Autodesk Inventor part; units mm, degrees
(part 2 of 2)
  line L683 (13.8193, -16.6595) -> (13.4103, -17.1969)
  line L684 (13.4103, -17.1969) -> (13.0544, -17.8466)
  line L685 (13.0544, -17.8466) -> (12.7817, -18.5147)
  line L686 (12.7817, -18.5147) -> (12.6178, -19.1068)
  line L687 (12.6178, -19.1068) -> (12.5603, -19.6314)
  line L688 (12.5603, -19.6314) -> (12.6069, -20.0971)
  line L689 (12.6069, -20.0971) -> (12.7553, -20.5124)
  line L690 (12.7553, -20.5124) -> (13.0032, -20.8859)
  line L691 (13.0032, -20.8859) -> (13.3484, -21.2261)
  line L692 (13.3484, -21.2261) -> (13.7885, -21.5415)
  line L693 (13.7885, -21.5415) -> (16.5319, -23.0238)
  line L694 (16.5319, -23.0238) -> (20.3466, -25.1761)
  line L695 (20.3466, -25.1761) -> (20.6486, -25.4525)
  line L696 (20.6486, -25.4525) -> (20.8116, -25.7931)
  line L697 (20.8116, -25.7931) -> (20.8459, -26.1675)
  line L698 (20.8459, -26.1675) -> (20.7618, -26.5456)
  line L699 (20.7618, -26.5456) -> (20.5697, -26.8968)
  line L700 (20.5697, -26.8968) -> (20.2799, -27.1909)
  line L701 (20.2799, -27.1909) -> (19.9026, -27.3974)
  line L702 (19.9026, -27.3974) -> (19.4483, -27.4862)
  line L703 (19.4483, -27.4862) -> (17.3984, -27.5067)
  line L704 (17.3984, -27.5067) -> (16.3264, -27.4862)
  line L705 (16.3264, -27.4862) -> (16.0758, -27.4173)
  line L706 (16.0758, -27.4173) -> (15.8933, -27.2387)
  line L707 (15.8933, -27.2387) -> (15.8038, -26.9924)
  line L708 (15.8038, -26.9924) -> (15.8323, -26.7206)
  line L709 (15.8323, -26.7206) -> (15.8735, -26.4369)
  line L710 (15.8735, -26.4369) -> (15.7983, -26.1616)
  line L711 (15.7983, -26.1616) -> (15.592, -25.9517)
  line L712 (15.592, -25.9517) -> (15.2394, -25.864)
  line L713 (15.2394, -25.864) -> (11.0542, -25.864)
  line L714 (11.0542, -25.864) -> (10.6479, -25.9075)
  line L715 (10.6479, -25.9075) -> (10.3167, -26.0305)
  line L716 (10.3167, -26.0305) -> (10.0596, -26.2215)
  line L717 (10.0596, -26.2215) -> (9.8757, -26.4694)
  line L718 (9.8757, -26.4694) -> (9.764, -26.7626)
  line L719 (9.764, -26.7626) -> (9.7235, -27.0899)
  line L720 (9.7235, -27.0899) -> (9.7533, -27.4399)
  line L721 (9.7533, -27.4399) -> (9.8525, -27.8013)
  line L722 (9.8525, -27.8013) -> (10.0202, -28.1626)
  line L723 (10.0202, -28.1626) -> (10.2553, -28.5126)
  line L724 (10.2553, -28.5126) -> (10.5569, -28.8399)
  line L725 (10.5569, -28.8399) -> (10.9242, -29.1332)
  line L726 (10.9242, -29.1332) -> (11.356, -29.381)
  line L727 (11.356, -29.381) -> (11.8516, -29.5721)
  line L728 (11.8516, -29.5721) -> (12.4099, -29.6951)
  line L729 (12.4099, -29.6951) -> (13.03, -29.7386)
  line L730 (13.03, -29.7386) -> (21.965, -29.7386)
  line L731 (21.965, -29.7386) -> (22.6253, -29.702)
  line L732 (22.6253, -29.702) -> (23.2336, -29.5897)
  line L733 (23.2336, -29.5897) -> (23.7942, -29.3979)
  line L734 (23.7942, -29.3979) -> (24.3112, -29.1228)
  line L735 (24.3112, -29.1228) -> (24.7889, -28.7605)
  line L736 (24.7889, -28.7605) -> (25.2316, -28.3073)
  line L737 (25.2316, -28.3073) -> (25.6435, -27.7593)
  line L738 (25.6435, -27.7593) -> (26.0289, -27.1127)
  line L739 (26.0289, -27.1127) -> (26.4193, -26.2607)
  line L740 (26.4193, -26.2607) -> (26.6201, -25.5322)
  line L741 (26.6201, -25.5322) -> (26.6506, -24.9094)
  line L742 (26.6506, -24.9094) -> (26.5304, -24.3745)
  line L743 (26.5304, -24.3745) -> (26.2786, -23.9096)
  line L744 (26.2786, -23.9096) -> (25.9146, -23.4968)
  line L745 (25.9146, -23.4968) -> (25.4579, -23.1183)
  line L746 (25.4579, -23.1183) -> (24.9277, -22.7562)
  line L747 (35.8308, -12.5417) -> (35.6711, -12.3549)
  line L748 (35.6711, -12.3549) -> (35.4659, -12.2167)
  line L749 (35.4659, -12.2167) -> (34.9498, -12.1015)
  line L750 (34.9498, -12.1015) -> (12.9562, -12.1015)
  line L751 (12.9562, -12.1015) -> (12.48, -12.1781)
  line L752 (12.48, -12.1781) -> (12.03, -12.39)
  line L753 (12.03, -12.39) -> (11.6489, -12.7098)
  line L754 (11.6489, -12.7098) -> (11.3795, -13.1102)
  line L755 (11.3795, -13.1102) -> (2.0043, -33.4309)
  line L756 (2.0043, -33.4309) -> (1.8927, -33.9479)
  line L757 (1.8927, -33.9479) -> (1.9323, -34.1923)
  line L758 (1.9323, -34.1923) -> (2.0351, -34.4159)
  line L759 (2.0351, -34.4159) -> (2.1948, -34.6028)
  line L760 (2.1948, -34.6028) -> (2.4002, -34.7412)
  line L761 (2.4002, -34.7412) -> (2.9168, -34.8567)
  line L762 (2.9168, -34.8567) -> (24.9341, -34.8567)
  line L763 (24.9341, -34.8567) -> (25.4106, -34.7799)
  line L764 (25.4106, -34.7799) -> (25.8605, -34.5676)
  line L765 (25.8605, -34.5676) -> (26.2412, -34.2474)
  line L766 (26.2412, -34.2474) -> (26.5102, -33.8467)
  line L767 (26.5102, -33.8467) -> (28.1619, -30.2583)
  line L768 (28.1619, -30.2583) -> (27.8028, -29.9601)
  line L769 (27.8028, -29.9601) -> (27.5106, -29.5935)
  line L770 (27.5106, -29.5935) -> (27.4336, -29.462)
  line L771 (27.4336, -29.462) -> (26.3715, -31.7689)
  line L772 (26.3715, -31.7689) -> (3.8665, -31.7689)
  line L773 (3.8665, -31.7689) -> (12.2831, -13.5267)
  line L774 (12.2831, -13.5267) -> (12.2831, -13.526)
  line L775 (12.2831, -13.526) -> (12.482, -13.0955)
  line L776 (12.482, -13.0955) -> (34.9498, -13.0955)
  line L777 (34.9498, -13.0955) -> (34.9639, -13.0968)
  line L778 (34.9639, -13.0968) -> (34.9594, -13.1109)
  line L779 (34.9594, -13.1109) -> (32.7699, -17.8684)
  line L780 (32.7699, -17.8684) -> (33.3832, -17.6303)
  line L781 (33.3832, -17.6303) -> (34.036, -17.4956)
  line L782 (34.036, -17.4956) -> (35.8629, -13.5267)
  line L783 (35.8629, -13.5267) -> (35.9739, -13.0094)
  line L784 (35.9739, -13.0094) -> (35.934, -12.765)
  line L785 (35.934, -12.765) -> (35.8308, -12.5417)
  point P0 (100, -50)
  point P1 (43.169, -21.3602)
  point P2 (43.426, -20.7976)
  point P3 (38.2792, -20.4356)
  point P4 (38.4651, -20.5971)
  point P5 (44.1555, -29.7302)
  constraints: 1572 end point, 1 point on line
sketch "Sketch17" plane through (-58, 50, -100) normal (-1, 0, 0) x (0, 0, 1)
  arc A0 (155.5169, -13.1936) -> (147.9671, -13.2014) centre (177.9783, -25519.1247) ccw
  arc A1 (164.0422, -13.1874) -> (155.5169, -13.1936) centre (180.5222, -28431.0385) ccw
  arc A2 (172.4068, -13.1839) -> (164.0422, -13.1874) centre (179.3768, -26483.535) ccw
  line L0 (172.4068, -13.1839) -> (192.49, -13.1786)
  line L1 (192.49, -13.1786) -> (192.4714, -13.7779)
  arc A3 (192.4714, -13.7779) -> (192.463, -14.0923) centre (229.4243, -14.9268) ccw
  arc A4 (192.463, -14.0923) -> (192.4526, -14.5768) centre (388.1411, -18.5105) ccw
  arc A5 (192.4526, -14.5768) -> (192.4423, -15.1225) centre (411.7864, -18.9861) ccw
  arc A6 (192.4423, -15.1225) -> (192.4336, -15.6562) centre (393.0535, -18.6562) ccw
  arc A7 (192.4247, -16.1476) -> (192.4336, -15.6562) centre (117.8838, -14.5414) ccw
  arc A8 (192.4135, -16.5636) -> (192.4247, -16.1476) centre (153.9256, -15.3181) ccw
  arc A9 (192.4012, -16.933) -> (192.4135, -16.5636) centre (-72.1561, -8.0018) ccw
  arc A10 (192.3918, -16.9493) -> (192.4012, -16.933) centre (192.3813, -16.9323) ccw
  arc A11 (192.3716, -16.9551) -> (192.3918, -16.9493) centre (192.3711, -16.9157) ccw
  arc A12 (191.4025, -16.9687) -> (192.3716, -16.9551) centre (85.6627, 7554.4624) ccw
  arc A13 (190.3279, -16.9824) -> (191.4025, -16.9687) centre (185.5858, 399.5447) ccw
  arc A14 (189.0559, -16.9958) -> (190.3279, -16.9824) centre (181.0678, 796.3096) ccw
  line L2 (189.0559, -16.9958) -> (185.7427, -17.0284)
  line L3 (185.7427, -17.0284) -> (184.3599, -17.8038)
  arc A15 (183.8287, -18.1011) -> (184.3599, -17.8038) centre (-6.9765, 323.4154) ccw
  arc A16 (183.3793, -18.3514) -> (183.8287, -18.1011) centre (86.1277, 156.7717) ccw
  arc A17 (182.9739, -18.5765) -> (183.3793, -18.3514) centre (-1472.0251, 2962.5768) ccw
  arc A18 (182.9636, -18.5792) -> (182.9739, -18.5765) centre (182.9636, -18.558) ccw
  arc A19 (182.9533, -18.5766) -> (182.9636, -18.5792) centre (182.9636, -18.5575) ccw
  arc A20 (182.535, -18.3501) -> (182.9533, -18.5766) centre (1951.8004, 3249.2088) ccw
  arc A21 (182.0715, -18.0984) -> (182.535, -18.3501) centre (284.7979, 170.5134) ccw
  arc A22 (181.5235, -17.7994) -> (182.0715, -18.0984) centre (382.7242, 350.3106) ccw
  line L4 (181.5235, -17.7994) -> (180.0969, -17.0197)
  line L5 (180.0969, -17.0197) -> (160.1888, -17.0208)
  arc A23 (160.1888, -17.0208) -> (144.3749, -17.0268) centre (161.6341, -24881.6326) ccw
  arc A24 (144.3749, -17.0268) -> (136.8231, -17.0497) centre (145.4933, -1626.5302) ccw
  arc A25 (136.8231, -17.0497) -> (132.0963, -17.0846) centre (143.2266, -1205.9023) ccw
  arc A26 (132.0963, -17.0846) -> (131.0777, -17.1776) centre (132.155, -23.3486) ccw
  arc A27 (131.0777, -17.1776) -> (130.7549, -17.273) centre (131.3311, -18.6291) ccw
  arc A28 (130.7549, -17.273) -> (130.46, -17.4396) centre (131.3448, -18.6615) ccw
  arc A29 (130.46, -17.4396) -> (130.2164, -17.663) centre (131.3024, -18.6028) ccw
  arc A30 (130.2164, -17.663) -> (130.0444, -17.9258) centre (131.1049, -18.4319) ccw
  arc A31 (130.0444, -17.9258) -> (129.9153, -18.3085) centre (131.5687, -18.6533) ccw
  arc A32 (129.9153, -18.3085) -> (129.8325, -18.8421) centre (135.0438, -19.3779) ccw
  arc A33 (129.8325, -18.8421) -> (129.791, -19.5222) centre (137.9858, -19.6803) ccw
  arc A34 (129.791, -19.5222) -> (129.7932, -20.3697) centre (149.1997, -19.8967) ccw
  arc A35 (129.7932, -20.3697) -> (129.8114, -20.9203) centre (161.1402, -19.6056) ccw
  arc A36 (129.8114, -20.9203) -> (129.8371, -21.2992) centre (137.1928, -20.6105) ccw
  arc A37 (129.8371, -21.2992) -> (129.8752, -21.5913) centre (133.8851, -20.9202) ccw
  arc A38 (129.8752, -21.5913) -> (129.932, -21.8528) centre (132.6128, -21.1331) ccw
  arc A39 (129.932, -21.8528) -> (130.0762, -22.1968) centre (131.2735, -21.4927) ccw
  arc A40 (130.0762, -22.1968) -> (130.3004, -22.4677) centre (131.0286, -21.6367) ccw
  arc A41 (130.3004, -22.4677) -> (130.6022, -22.658) centre (131.0525, -21.6094) ccw
  arc A42 (130.6022, -22.658) -> (130.9734, -22.7654) centre (131.2185, -21.223) ccw
  arc A43 (130.9734, -22.7654) -> (131.5045, -22.8166) centre (131.6549, -18.476) ccw
  arc A44 (131.5045, -22.8166) -> (132.8291, -22.855) centre (135.5677, 94.4652) ccw
  arc A45 (132.8291, -22.855) -> (134.8809, -22.8934) centre (138.0008, 198.702) ccw
  arc A46 (134.8809, -22.8934) -> (138.4757, -22.9405) centre (161.0223, 1833.8913) ccw
  arc A47 (141.0206, -22.9772) -> (138.4757, -22.9405) centre (131.717, -579.5957) ccw
  arc A48 (142.6378, -23.0177) -> (141.0206, -22.9772) centre (139.3924, -120.3907) ccw
  arc A49 (143.7571, -23.0692) -> (142.6378, -23.0177) centre (141.1689, -67.087) ccw
  arc A50 (144.5556, -23.1431) -> (143.7571, -23.0692) centre (143.0556, -34.9983) ccw
  arc A51 (145.317, -23.2838) -> (144.5556, -23.1431) centre (143.701, -29.8979) ccw
  arc A52 (146.093, -23.5149) -> (145.317, -23.2838) centre (143.3852, -31.1905) ccw
  arc A53 (146.8189, -23.8134) -> (146.093, -23.5149) centre (143.5298, -30.7805) ccw
  arc A54 (147.4285, -24.1566) -> (146.8189, -23.8134) centre (144.7359, -28.2256) ccw
  arc A55 (147.7255, -24.3826) -> (147.4285, -24.1566) centre (145.8661, -26.5177) ccw
  arc A56 (148.0655, -24.7) -> (147.7255, -24.3826) centre (143.2906, -29.4751) ccw
  arc A57 (148.383, -25.0401) -> (148.0655, -24.7) centre (143.2904, -29.4753) ccw
  arc A58 (148.609, -25.3371) -> (148.383, -25.0401) centre (146.2466, -26.9007) ccw
  arc A59 (148.9308, -25.9) -> (148.609, -25.3371) centre (144.4706, -28.0761) ccw
  arc A60 (149.1657, -26.484) -> (148.9308, -25.9) centre (144.9676, -27.8336) ccw
  arc A61 (149.3254, -27.126) -> (149.1657, -26.484) centre (144.4771, -27.9913) ccw
  arc A62 (149.4214, -27.8641) -> (149.3254, -27.126) centre (141.5782, -28.5088) ccw
  arc A63 (149.4533, -28.4552) -> (149.4214, -27.8641) centre (138.9674, -28.7233) ccw
  arc A64 (149.4702, -29.3971) -> (149.4533, -28.4552) centre (87.0184, -30.052) ccw
  arc A65 (149.4733, -30.3333) -> (149.4702, -29.3971) centre (84.3091, -30.0805) ccw
  arc A66 (149.4529, -30.8676) -> (149.4733, -30.3333) centre (141.6731, -30.3031) ccw
  arc A67 (149.3251, -31.9543) -> (149.4529, -30.8676) centre (137.2306, -29.9807) ccw
  arc A68 (149.1085, -32.8875) -> (149.3251, -31.9543) centre (142.1906, -30.7901) ccw
  arc A69 (148.8006, -33.6818) -> (149.1085, -32.8875) centre (143.7022, -31.2484) ccw
  arc A70 (148.3967, -34.35) -> (148.8006, -33.6818) centre (145.2104, -31.9682) ccw
  arc A71 (147.9836, -34.8205) -> (148.3967, -34.35) centre (145.2057, -31.9647) ccw
  arc A72 (147.4851, -35.2416) -> (147.9836, -34.8205) centre (144.7342, -31.48) ccw
  arc A73 (146.9055, -35.6091) -> (147.4851, -35.2416) centre (144.4327, -31.0677) ccw
  arc A74 (146.2491, -35.9202) -> (146.9055, -35.6091) centre (143.8047, -29.9143) ccw
  arc A75 (145.5174, -36.1782) -> (146.2491, -35.9202) centre (143.1741, -28.3651) ccw
  arc A76 (144.8818, -36.3144) -> (145.5174, -36.1782) centre (144.3529, -32.2955) ccw
  arc A77 (144.0427, -36.3836) -> (144.8818, -36.3144) centre (143.7489, -27.7054) ccw
  arc A78 (142.4034, -36.4263) -> (144.0427, -36.3836) centre (140.5007, 68.2463) ccw
  arc A79 (140.1178, -36.4532) -> (142.4034, -36.4263) centre (139.1652, 141.7316) ccw
  arc A80 (133.2261, -36.4874) -> (140.1178, -36.4532) centre (92.1448, 8937.0184) ccw
  arc A81 (125.4771, -36.5228) -> (133.2261, -36.4874) centre (-2083.9915, 484275.8678) ccw
  arc A82 (125.4315, -36.504) -> (125.4771, -36.5228) centre (125.4768, -36.4586) ccw
  arc A83 (125.4001, -36.4199) -> (125.4315, -36.504) centre (125.5079, -36.4276) ccw
  arc A84 (125.5112, -34.8712) -> (125.4001, -36.4199) centre (1139.0305, -108.3625) ccw
  arc A85 (125.6207, -33.4758) -> (125.5112, -34.8712) centre (242.9379, -43.3859) ccw
  arc A86 (125.7137, -32.6116) -> (125.6207, -33.4758) centre (144.5147, -35.0719) ccw
  line L6 (125.7137, -32.6116) -> (125.7463, -32.3629)
  line L7 (125.7463, -32.3629) -> (128.0606, -32.344)
  arc A87 (129.233, -32.3348) -> (128.0606, -32.344) centre (143.2898, -1899.2591) ccw
  arc A88 (130.9251, -32.3222) -> (129.233, -32.3348) centre (188.2055, -7866.3318) ccw
  arc A89 (132.7895, -32.3088) -> (130.9251, -32.3222) centre (194.025, -8663.7021) ccw
  arc A90 (134.5625, -32.2964) -> (132.7895, -32.3088) centre (182.7017, -7067.7613) ccw
  arc A91 (134.5625, -32.2964) -> (137.764, -32.2708) centre (125.0883, 1352.4691) ccw
  arc A92 (137.764, -32.2708) -> (140.2452, -32.2421) centre (133.1173, 475.3515) ccw
  arc A93 (140.2452, -32.2421) -> (142.1303, -32.2115) centre (134.1053, 404.949) ccw
  arc A94 (142.1303, -32.2115) -> (142.8794, -32.1797) centre (141.8456, -16.7006) ccw
  arc A95 (142.8794, -32.1797) -> (143.3579, -32.1351) centre (142.2685, -23.0334) ccw
  arc A96 (143.3579, -32.1351) -> (143.6523, -32.0701) centre (143.175, -30.6069) ccw
  arc A97 (143.6523, -32.0701) -> (143.8804, -31.9604) centre (143.3561, -31.1621) ccw
  arc A98 (143.8804, -31.9604) -> (144.1182, -31.7755) centre (142.8417, -30.3788) ccw
  arc A99 (144.1182, -31.7755) -> (144.3129, -31.559) centre (143.1141, -30.6768) ccw
  arc A100 (144.3129, -31.559) -> (144.4604, -31.31) centre (143.1418, -30.6972) ccw
  arc A101 (144.4604, -31.31) -> (144.5686, -31.0105) centre (142.8242, -30.5497) ccw
  arc A102 (144.5686, -31.0105) -> (144.6452, -30.6414) centre (141.1655, -30.1114) ccw
  arc A103 (144.6452, -30.6414) -> (144.6784, -30.2514) centre (141.7211, -30.1961) ccw
  arc A104 (144.6784, -30.2514) -> (144.6793, -29.6224) centre (126.4761, -29.9106) ccw
  arc A105 (144.6793, -29.6224) -> (144.6584, -28.9933) centre (126.5363, -29.9096) ccw
  arc A106 (144.6584, -28.9933) -> (144.6129, -28.6006) centre (141.6144, -29.1472) ccw
  arc A107 (144.6129, -28.6006) -> (144.5174, -28.176) centre (139.3813, -29.5543) ccw
  arc A108 (144.5174, -28.176) -> (144.3964, -27.814) centre (141.4643, -28.9953) ccw
  arc A109 (144.3964, -27.814) -> (144.2589, -27.5316) centre (142.3172, -28.6517) ccw
  arc A110 (144.2589, -27.5316) -> (144.1126, -27.3587) centre (143.7081, -27.8493) ccw
  arc A111 (144.1126, -27.3587) -> (143.9773, -27.2622) centre (143.3558, -28.2767) ccw
  arc A112 (143.9773, -27.2622) -> (143.8134, -27.1727) centre (142.9904, -28.8733) ccw
  arc A113 (143.8134, -27.1727) -> (143.6348, -27.0965) centre (142.9305, -28.997) ccw
  arc A114 (143.6348, -27.0965) -> (143.4547, -27.0403) centre (143.0072, -28.7903) ccw
  arc A115 (143.4547, -27.0403) -> (142.8088, -26.9349) centre (142.5385, -30.6227) ccw
  arc A116 (142.8088, -26.9349) -> (141.6227, -26.8682) centre (140.258, -61.7364) ccw
  arc A117 (141.6227, -26.8682) -> (139.7603, -26.8159) centre (138.31, -111.5069) ccw
  arc A118 (139.7603, -26.8159) -> (136.4685, -26.7669) centre (127.2442, -757.6481) ccw
  arc A119 (132.1738, -26.7016) -> (136.4685, -26.7669) centre (146.966, 804.9237) ccw
  arc A120 (130.1637, -26.6258) -> (132.1738, -26.7016) centre (133.0723, 23.8123) ccw
  arc A121 (128.962, -26.5051) -> (130.1637, -26.6258) centre (130.9817, -12.4402) ccw
  arc A122 (128.1426, -26.2868) -> (128.962, -26.5051) centre (129.475, -22.9325) ccw
  arc A123 (127.8662, -26.1658) -> (128.1426, -26.2868) centre (129.7587, -22.2183) ccw
  arc A124 (127.5074, -25.9871) -> (127.8662, -26.1658) centre (133.644, -14.1144) ccw
  arc A125 (127.1584, -25.8001) -> (127.5074, -25.9871) centre (133.6434, -14.1154) ccw
  arc A126 (126.9188, -25.6542) -> (127.1584, -25.8001) centre (128.8501, -22.7519) ccw
  arc A127 (126.1599, -25.0036) -> (126.9188, -25.6542) centre (129.203, -22.2216) ccw
  arc A128 (125.5888, -24.1958) -> (126.1599, -25.0036) centre (129.0808, -22.3334) ccw
  arc A129 (125.1908, -23.1929) -> (125.5888, -24.1958) centre (129.8432, -21.9267) ccw
  arc A130 (124.9475, -21.9581) -> (125.1908, -23.1929) centre (133.7282, -20.8694) ccw
  arc A131 (124.8648, -20.9473) -> (124.9475, -21.9581) centre (136.9954, -20.4643) ccw
  arc A132 (124.8512, -19.7875) -> (124.8648, -20.9473) centre (145.5578, -20.1234) ccw
  arc A133 (124.9018, -18.6484) -> (124.8512, -19.7875) centre (145.0731, -20.1155) ccw
  arc A134 (125.0165, -17.7049) -> (124.9018, -18.6484) centre (134.7063, -19.3615) ccw
  arc A135 (125.4488, -16.1894) -> (125.0165, -17.7049) centre (132.1861, -18.9306) ccw
  arc A136 (126.1616, -15.0517) -> (125.4488, -16.1894) centre (129.055, -17.6567) ccw
  arc A137 (127.2203, -14.2215) -> (126.1616, -15.0517) centre (129.0698, -17.6701) ccw
  arc A138 (128.6884, -13.6265) -> (127.2203, -14.2215) centre (130.7167, -20.7407) ccw
  arc A139 (129.1047, -13.5188) -> (128.6884, -13.6265) centre (131.1038, -22.0988) ccw
  arc A140 (129.5379, -13.428) -> (129.1047, -13.5188) centre (131.3473, -23.1438) ccw
  arc A141 (129.9544, -13.3604) -> (129.5379, -13.428) centre (131.2044, -22.3763) ccw
  arc A142 (130.3189, -13.3229) -> (129.9544, -13.3604) centre (130.6687, -18.5128) ccw
  arc A143 (131.4135, -13.2778) -> (130.3189, -13.3229) centre (131.7298, -34.2563) ccw
  arc A144 (133.8397, -13.2488) -> (131.4135, -13.2778) centre (137.2898, -403.0703) ccw
  arc A145 (137.4318, -13.2263) -> (133.8397, -13.2488) centre (139.9441, -702.9681) ccw
  arc A146 (143.1109, -13.2097) -> (137.4318, -13.2263) centre (152.0364, -4023.8902) ccw
  arc A147 (147.9671, -13.2014) -> (143.1109, -13.2097) centre (153.4228, -4646.9534) ccw
  arc A148 (160.2515, -18.4737) -> (156.129, -18.4661) centre (156.7117, -819.255) ccw
  arc A149 (164.3509, -18.5017) -> (160.2515, -18.4737) centre (156.4702, -873.9576) ccw
  arc A150 (166.5605, -18.5512) -> (164.3509, -18.5017) centre (163.5792, -102.2694) ccw
  arc A151 (167.1372, -18.5774) -> (166.5605, -18.5512) centre (165.5149, -47.9138) ccw
  arc A152 (167.5467, -18.6109) -> (167.1372, -18.5774) centre (166.7067, -26.3617) ccw
  arc A153 (167.9004, -18.661) -> (167.5467, -18.6109) centre (166.9566, -24.0562) ccw
  arc A154 (168.2865, -18.7382) -> (167.9004, -18.661) centre (166.5107, -26.6048) ccw
  arc A155 (169.3046, -19.0709) -> (168.2865, -18.7382) centre (167.0269, -24.318) ccw
  arc A156 (170.0804, -19.5557) -> (169.3046, -19.0709) centre (168.0778, -21.8972) ccw
  arc A157 (170.6597, -20.2318) -> (170.0804, -19.5557) centre (168.2032, -21.7505) ccw
  arc A158 (171.0898, -21.1358) -> (170.6597, -20.2318) centre (166.7717, -22.6355) ccw
  arc A159 (171.2294, -21.6476) -> (171.0898, -21.1358) centre (167.3979, -22.418) ccw
  arc A160 (171.3016, -22.183) -> (171.2294, -21.6476) centre (167.1089, -22.4761) ccw
  arc A161 (171.3331, -22.9899) -> (171.3016, -22.183) centre (158.2198, -23.0977) ccw
  arc A162 (171.3405, -24.7218) -> (171.3331, -22.9899) centre (-47.671, -24.7899) ccw
  arc A163 (171.3337, -26.523) -> (171.3405, -24.7218) centre (-49.4983, -24.7902) ccw
  arc A164 (171.2977, -27.2892) -> (171.3337, -26.523) centre (161.5297, -26.4461) ccw
  arc A165 (171.209, -27.7966) -> (171.2977, -27.2892) centre (168.3429, -27.0342) ccw
  arc A166 (171.0306, -28.3118) -> (171.209, -27.7966) centre (167.6154, -26.8407) ccw
  arc A167 (170.7093, -28.9398) -> (171.0306, -28.3118) centre (166.1313, -26.2014) ccw
  arc A168 (170.3469, -29.4226) -> (170.7093, -28.9398) centre (168.2347, -27.4595) ccw
  arc A169 (169.9033, -29.8061) -> (170.3469, -29.4226) centre (168.3751, -27.59) ccw
  arc A170 (169.3377, -30.1333) -> (169.9033, -29.8061) centre (167.5588, -26.4064) ccw
  arc A171 (169.0516, -30.2578) -> (169.3377, -30.1333) centre (167.4111, -26.0969) ccw
  arc A172 (168.7171, -30.3807) -> (169.0516, -30.2578) centre (166.2723, -23.2085) ccw
  arc A173 (168.3968, -30.4816) -> (168.7171, -30.3807) centre (166.3933, -23.5635) ccw
  arc A174 (168.1644, -30.5333) -> (168.3968, -30.4816) centre (167.8718, -28.6689) ccw
  arc A175 (167.8348, -30.5709) -> (168.1644, -30.5333) centre (167.5494, -26.6139) ccw
  arc A176 (167.3299, -30.601) -> (167.8348, -30.5709) centre (166.3793, -10.3912) ccw
  arc A177 (166.6383, -30.627) -> (167.3299, -30.601) centre (165.6256, 5.6323) ccw
  arc A178 (165.6773, -30.6503) -> (166.6383, -30.627) centre (162.9825, 100.2759) ccw
  arc A179 (164.209, -30.6735) -> (165.6773, -30.6503) centre (162.4802, 124.6803) ccw
  arc A180 (161.2231, -30.7047) -> (164.209, -30.6735) centre (140.0602, 2139.3547) ccw
  arc A181 (158.2383, -30.7317) -> (161.2231, -30.7047) centre (140.7828, 2065.3292) ccw
  arc A182 (156.6918, -30.7379) -> (158.2383, -30.7317) centre (156.7484, 148.1768) ccw
  line L8 (156.6918, -30.7379) -> (156.0059, -30.7377)
  line L9 (156.0059, -30.7377) -> (156.0059, -36.5137)
  line L10 (156.0059, -36.5137) -> (152.3959, -36.5137)
  line L11 (152.3959, -36.5137) -> (152.3967, -30.4128)
  arc A183 (152.4026, -26.182) -> (152.3967, -30.4128) centre (1815.4435, -30.6335) ccw
  arc A184 (152.4195, -22.4306) -> (152.4026, -26.182) centre (1181.8899, -28.9392) ccw
  arc A185 (152.4421, -19.1057) -> (152.4195, -22.4306) centre (3587.1631, -44.1483) ccw
  arc A186 (152.4708, -18.6949) -> (152.4421, -19.1057) centre (155.7493, -19.1299) ccw
  arc A187 (152.4838, -18.6163) -> (152.4708, -18.6949) centre (153.69, -18.8567) ccw
  arc A188 (152.4994, -18.5733) -> (152.4838, -18.6163) centre (152.6328, -18.646) ccw
  arc A189 (152.5229, -18.548) -> (152.4994, -18.5733) centre (152.5609, -18.6069) ccw
  arc A190 (152.5595, -18.5321) -> (152.5229, -18.548) centre (152.5893, -18.6507) ccw
  arc A191 (152.6118, -18.5245) -> (152.5595, -18.5321) centre (152.6222, -18.7817) ccw
  arc A192 (152.8946, -18.5137) -> (152.6118, -18.5245) centre (155.6961, -95.1113) ccw
  arc A193 (153.2245, -18.5031) -> (152.8946, -18.5137) centre (154.2093, -54.4605) ccw
  arc A194 (153.6026, -18.4939) -> (153.2245, -18.5031) centre (154.919, -80.3692) ccw
  arc A195 (156.129, -18.4661) -> (153.6026, -18.4939) centre (156.2185, -141.4519) ccw
  arc A196 (163.9717, -22.1247) -> (161.9831, -22.1028) centre (157.1642, -548.2186) ccw
  arc A197 (165.3347, -22.15) -> (163.9717, -22.1247) centre (162.4024, -143.3926) ccw
  arc A198 (166.2928, -22.18) -> (165.3347, -22.15) centre (163.7001, -89.7313) ccw
  arc A199 (166.8202, -22.2198) -> (166.2928, -22.18) centre (166.0175, -29.3523) ccw
  arc A200 (167.0243, -22.2535) -> (166.8202, -22.2198) centre (166.5963, -24.2092) ccw
  arc A201 (167.1823, -22.3048) -> (167.0243, -22.2535) centre (166.8438, -23.0783) ccw
  arc A202 (167.3197, -22.3832) -> (167.1823, -22.3048) centre (166.882, -22.9909) ccw
  arc A203 (167.4596, -22.4996) -> (167.3197, -22.3832) centre (166.5587, -23.4399) ccw
  arc A204 (167.5682, -22.6253) -> (167.4596, -22.4996) centre (166.8489, -23.1369) ccw
  arc A205 (167.6557, -22.7734) -> (167.5682, -22.6253) centre (166.7399, -23.2145) ccw
  arc A206 (167.7249, -22.95) -> (167.6557, -22.7734) centre (166.5247, -23.3181) ccw
  arc A207 (167.7782, -23.1612) -> (167.7249, -22.95) centre (165.6442, -23.5883) ccw
  arc A208 (167.8382, -23.7012) -> (167.7782, -23.1612) centre (164.7086, -23.7755) ccw
  arc A209 (167.8516, -24.8334) -> (167.8382, -23.7012) centre (120.5368, -24.8244) ccw
  arc A210 (167.839, -25.9707) -> (167.8516, -24.8334) centre (115.5533, -24.8234) ccw
  arc A211 (167.7776, -26.4462) -> (167.839, -25.9707) centre (165.5819, -25.9211) ccw
  arc A212 (167.6979, -26.6957) -> (167.7776, -26.4462) centre (166.0693, -26.0377) ccw
  arc A213 (167.592, -26.88) -> (167.6979, -26.6957) centre (166.9785, -26.405) ccw
  arc A214 (167.4378, -27.0321) -> (167.592, -26.88) centre (166.9485, -26.3818) ccw
  arc A215 (167.2078, -27.1823) -> (167.4378, -27.0321) centre (166.1985, -25.385) ccw
  arc A216 (167.0247, -27.2617) -> (167.2078, -27.1823) centre (166.7301, -26.3317) ccw
  arc A217 (166.7997, -27.3169) -> (167.0247, -27.2617) centre (166.4938, -25.5856) ccw
  arc A218 (166.4952, -27.3565) -> (166.7997, -27.3169) centre (166.2141, -24.0022) ccw
  arc A219 (166.0494, -27.3869) -> (166.4952, -27.3565) centre (165.2875, -12.9471) ccw
  arc A220 (165.3966, -27.409) -> (166.0494, -27.3869) centre (165.1392, -10.1383) ccw
  arc A221 (163.4693, -27.4354) -> (165.3966, -27.409) centre (153.2679, 786.4653) ccw
  arc A222 (161.0365, -27.462) -> (163.4693, -27.4354) centre (154.0239, 726.2122) ccw
  arc A223 (158.0636, -27.487) -> (161.0365, -27.462) centre (145.5307, 1638.9805) ccw
  line L12 (158.0636, -27.487) -> (156.0059, -27.5025)
  line L13 (156.0059, -27.5025) -> (156.0059, -22.0737)
  line L14 (156.0059, -22.0737) -> (157.4715, -22.0743)
  arc A224 (158.2361, -22.0763) -> (157.4715, -22.0743) centre (157.403, -190.189) ccw
  arc A225 (159.4014, -22.0829) -> (158.2361, -22.0763) centre (153.9901, -878.8931) ccw
  arc A226 (160.7094, -22.092) -> (159.4014, -22.0829) centre (153.3441, -981.0773) ccw
  arc A227 (161.9831, -22.1028) -> (160.7094, -22.092) centre (154.1006, -882.6539) ccw
  arc A228 (186.2041, -18.4737) -> (185.9487, -18.4853) centre (186.3916, -25.4207) ccw
  arc A229 (186.6401, -18.4671) -> (186.2041, -18.4737) centre (186.6998, -36.8335) ccw
  arc A230 (187.6006, -18.4653) -> (186.6401, -18.4671) centre (187.7294, -353.8358) ccw
  arc A231 (189.0313, -18.4723) -> (187.6006, -18.4653) centre (187.6529, -154.668) ccw
  arc A232 (189.9516, -18.4986) -> (189.0313, -18.4723) centre (188.7787, -43.4348) ccw
  arc A233 (190.5982, -18.5376) -> (189.9516, -18.4986) centre (188.7991, -42.9997) ccw
  arc A234 (190.7228, -18.6122) -> (190.5982, -18.5376) centre (190.5864, -18.6987) ccw
  arc A235 (190.7595, -18.7435) -> (190.7228, -18.6122) centre (190.523, -18.7389) ccw
  arc A236 (190.7308, -20.0994) -> (190.7595, -18.7435) centre (-251.767, -10.0433) ccw
  arc A237 (190.6942, -21.3367) -> (190.7308, -20.0994) centre (100.8949, -18.0578) ccw
  arc A238 (190.6451, -22.0349) -> (190.6942, -21.3367) centre (180.3171, -20.9578) ccw
  line L15 (190.6451, -22.0349) -> (190.6295, -22.1838)
  line L16 (190.6295, -22.1838) -> (185.0358, -22.1976)
  arc A239 (185.0358, -22.1976) -> (182.5259, -22.2056) centre (189.25, -1731.9185) ccw
  arc A240 (182.5259, -22.2056) -> (180.7079, -22.2162) centre (184.4275, -505.7265) ccw
  arc A241 (180.7079, -22.2162) -> (179.3571, -22.2285) centre (184.3308, -493.2072) ccw
  arc A242 (179.3571, -22.2285) -> (178.9366, -22.2445) centre (179.438, -29.8932) ccw
  arc A243 (178.9366, -22.2445) -> (178.3771, -22.2928) centre (179.8274, -35.8318) ccw
  arc A244 (178.3771, -22.2928) -> (177.9751, -22.3574) centre (178.7898, -26.1457) ccw
  arc A245 (177.9751, -22.3574) -> (177.6857, -22.4421) centre (178.4108, -24.3832) ccw
  arc A246 (177.6857, -22.4421) -> (177.4919, -22.5552) centre (177.9163, -23.0596) ccw
  arc A247 (177.4919, -22.5552) -> (177.4521, -22.597) centre (177.6619, -22.7572) ccw
  arc A248 (177.4521, -22.597) -> (177.4021, -22.6673) centre (178.4412, -23.3525) ccw
  arc A249 (177.4021, -22.6673) -> (177.3515, -22.7501) centre (178.5896, -23.4504) ccw
  arc A250 (177.3515, -22.7501) -> (177.3077, -22.8345) centre (178.4905, -23.3944) ccw
  arc A251 (177.3077, -22.8345) -> (177.2079, -23.0759) centre (179.6654, -23.9504) ccw
  arc A252 (177.2079, -23.0759) -> (177.1484, -23.2947) centre (178.6095, -23.5747) ccw
  arc A253 (177.1484, -23.2947) -> (177.1149, -23.5537) centre (179.2638, -23.7) ccw
  arc A254 (177.1149, -23.5537) -> (177.0966, -23.9364) centre (186.6128, -24.2005) ccw
  arc A255 (177.0966, -23.9364) -> (177.0959, -24.3495) centre (185.0107, -24.156) ccw
  arc A256 (177.0959, -24.3495) -> (177.121, -24.6727) centre (180.1377, -24.2752) ccw
  arc A257 (177.121, -24.6727) -> (177.1755, -24.9475) centre (179.2772, -24.3886) ccw
  arc A258 (177.1755, -24.9475) -> (177.2642, -25.2091) centre (179.1612, -24.4194) ccw
  arc A259 (177.2642, -25.2091) -> (177.4299, -25.5178) centre (178.9154, -24.5218) ccw
  arc A260 (177.4299, -25.5178) -> (177.6227, -25.7046) centre (177.9631, -25.1603) ccw
  arc A261 (177.6227, -25.7046) -> (177.9031, -25.8196) centre (178.0987, -24.9434) ccw
  arc A262 (177.9031, -25.8196) -> (178.3697, -25.9004) centre (178.9759, -21.0138) ccw
  arc A263 (178.3697, -25.9004) -> (178.9667, -25.9523) centre (179.3769, -17.7814) ccw
  arc A264 (178.9667, -25.9523) -> (179.9044, -25.9898) centre (181.2718, 19.961) ccw
  arc A265 (179.9044, -25.9898) -> (181.3291, -26.023) centre (183.1902, 84.4299) ccw
  arc A266 (181.3291, -26.023) -> (183.7307, -26.0599) centre (194.9275, 780.9511) ccw
  arc A267 (186.6484, -26.1084) -> (183.7307, -26.0599) centre (176.3425, -558.5143) ccw
  arc A268 (188.0813, -26.1632) -> (186.6484, -26.1084) centre (185.9127, -64.1124) ccw
  arc A269 (188.9703, -26.2486) -> (188.0813, -26.1632) centre (187.4229, -37.686) ccw
  arc A270 (189.6333, -26.3972) -> (188.9703, -26.2486) centre (188.4402, -30.1668) ccw
  arc A271 (190.1242, -26.5753) -> (189.6333, -26.3972) centre (187.7301, -32.4102) ccw
  arc A272 (190.5351, -26.7743) -> (190.1242, -26.5753) centre (188.7202, -29.9972) ccw
  arc A273 (190.9014, -27.0133) -> (190.5351, -26.7743) centre (188.8887, -29.698) ccw
  arc A274 (191.2569, -27.3115) -> (190.9014, -27.0133) centre (188.3537, -30.4115) ccw
  arc A275 (191.6981, -27.7909) -> (191.2569, -27.3115) centre (188.2511, -30.5211) ccw
  arc A276 (192.0155, -28.2865) -> (191.6981, -27.7909) centre (189.3929, -29.6167) ccw
  arc A277 (192.2355, -28.8491) -> (192.0155, -28.2865) centre (189.2271, -29.7008) ccw
  arc A278 (192.383, -29.5317) -> (192.2355, -28.8491) centre (186.8975, -30.3603) ccw
  arc A279 (192.423, -29.9432) -> (192.383, -29.5317) centre (188.5352, -30.113) ccw
  arc A280 (192.4438, -30.624) -> (192.423, -29.9432) centre (166.2553, -31.0857) ccw
  arc A281 (192.4464, -31.3449) -> (192.4438, -30.624) centre (166.7531, -31.077) ccw
  arc A282 (192.4255, -31.9397) -> (192.4464, -31.3449) centre (180.4317, -31.2196) ccw
  arc A283 (192.3089, -33.1136) -> (192.4255, -31.9397) centre (177.3399, -31.034) ccw
  arc A284 (192.1074, -33.9277) -> (192.3089, -33.1136) centre (188.3319, -32.5611) ccw
  arc A285 (191.7713, -34.5786) -> (192.1074, -33.9277) centre (189.4375, -32.9613) ccw
  arc A286 (191.2401, -35.2144) -> (191.7713, -34.5786) centre (187.9803, -31.9515) ccw
  arc A287 (190.8612, -35.5594) -> (191.2401, -35.2144) centre (187.3306, -31.3011) ccw
  arc A288 (190.5137, -35.803) -> (190.8612, -35.5594) centre (189.1855, -33.5384) ccw
  arc A289 (190.0958, -36.0106) -> (190.5137, -35.803) centre (188.808, -32.8947) ccw
  arc A290 (189.4778, -36.248) -> (190.0958, -36.0106) centre (185.0762, -23.8649) ccw
  line L17 (189.4778, -36.248) -> (188.9147, -36.4482)
  line L18 (188.9147, -36.4482) -> (181.3966, -36.4837)
  arc A291 (178.5128, -36.4963) -> (181.3966, -36.4837) centre (161.8205, 4106.8398) ccw
  arc A292 (176.0829, -36.5047) -> (178.5128, -36.4963) centre (170.0734, 2058.2955) ccw
  arc A293 (173.8784, -36.511) -> (176.0829, -36.5047) centre (-140.2231, 110186.1793) ccw
  arc A294 (173.8646, -36.5053) -> (173.8784, -36.511) centre (173.8784, -36.4916) ccw
  arc A295 (173.8462, -36.4562) -> (173.8646, -36.5053) centre (173.9094, -36.4605) ccw
  arc A296 (173.936, -35.1444) -> (173.8462, -36.4562) centre (1985.7675, -159.8181) ccw
  arc A297 (174.0207, -33.9791) -> (173.936, -35.1444) centre (323.2879, -45.4214) ccw
  arc A298 (174.084, -33.3173) -> (174.0207, -33.9791) centre (191.6694, -35.332) ccw
  arc A299 (174.084, -33.3173) -> (174.0952, -33.2163) centre (160.3888, -31.7482) ccw
  arc A300 (174.0952, -33.2163) -> (174.1047, -33.1235) centre (164.3772, -32.1754) ccw
  arc A301 (174.1047, -33.1235) -> (174.112, -33.0457) centre (163.3044, -32.0708) ccw
  arc A302 (174.112, -33.0457) -> (174.1134, -33.0154) centre (173.7558, -33.0136) ccw
  arc A303 (174.1547, -32.9734) -> (174.1134, -33.0154) centre (174.1556, -33.0156) ccw
  arc A304 (175.1113, -32.9543) -> (174.1547, -32.9734) centre (179.8019, -292.0874) ccw
  arc A305 (176.6417, -32.9337) -> (175.1113, -32.9543) centre (178.1037, -198.2757) ccw
  arc A306 (180.3373, -32.9027) -> (176.6417, -32.9337) centre (212.789, -4121.0029) ccw
  arc A307 (180.3373, -32.9027) -> (184.45, -32.8628) centre (171.0744, 1134.1611) ccw
  arc A308 (184.45, -32.8628) -> (186.451, -32.8151) centre (183.5253, 47.8189) ccw
  arc A309 (186.451, -32.8151) -> (187.6467, -32.7481) centre (185.347, -2.3896) ccw
  arc A310 (187.6467, -32.7481) -> (188.1616, -32.6188) centre (187.5285, -31.1878) ccw
  arc A311 (188.1616, -32.6188) -> (188.3248, -32.5094) centre (187.9319, -32.0996) ccw
  arc A312 (188.3248, -32.5094) -> (188.4658, -32.3371) centre (187.6849, -31.842) ccw
  arc A313 (188.4658, -32.3371) -> (188.5793, -32.1088) centre (187.4276, -31.6789) ccw
  arc A314 (188.5793, -32.1088) -> (188.6602, -31.8324) centre (186.7161, -31.4133) ccw
  arc A315 (188.6602, -31.8324) -> (188.704, -31.4892) centre (186.6732, -31.4041) ccw
  arc A316 (188.704, -31.4892) -> (188.7164, -30.914) centre (174.6149, -30.8986) ccw
  arc A317 (188.7164, -30.914) -> (188.7064, -30.3418) centre (173.3324, -30.8972) ccw
  arc A318 (188.7064, -30.3418) -> (188.6621, -30.0522) centre (187.4363, -30.3877) ccw
  arc A319 (188.6621, -30.0522) -> (188.6108, -29.8947) centre (186.9867, -30.5108) ccw
  arc A320 (188.6108, -29.8947) -> (188.5424, -29.7346) centre (186.6365, -30.6436) ccw
  arc A321 (188.5424, -29.7346) -> (188.4679, -29.5941) centre (186.8482, -30.5427) ccw
  arc A322 (188.4679, -29.5941) -> (188.3988, -29.5002) centre (187.9858, -29.8764) ccw
  arc A323 (188.3988, -29.5002) -> (188.3115, -29.4267) centre (188.0799, -29.7907) ccw
  arc A324 (188.3115, -29.4267) -> (188.1861, -29.3586) centre (187.757, -30.2983) ccw
  arc A325 (188.1861, -29.3586) -> (188.033, -29.2998) centre (187.6315, -30.5731) ccw
  arc A326 (188.033, -29.2998) -> (187.8605, -29.2543) centre (187.472, -31.0787) ccw
  arc A327 (187.8605, -29.2543) -> (187.2709, -29.1702) centre (186.9502, -33.5286) ccw
  arc A328 (187.2709, -29.1702) -> (186.3375, -29.1193) centre (185.4589, -53.7971) ccw
  arc A329 (186.3375, -29.1193) -> (184.749, -29.077) centre (183.1809, -117.7764) ccw
  arc A330 (184.749, -29.077) -> (181.247, -29.0189) centre (156.0335, -1653.3701) ccw
  arc A331 (179.5754, -28.9868) -> (181.247, -29.0189) centre (184.7781, 198.4893) ccw
  arc A332 (178.3058, -28.9473) -> (179.5754, -28.9868) centre (181.3411, 48.2199) ccw
  arc A333 (177.3608, -28.9012) -> (178.3058, -28.9473) centre (180.2884, 21.4573) ccw
  arc A334 (176.842, -28.8456) -> (177.3608, -28.9012) centre (177.6713, -23.5602) ccw
  arc A335 (176.4152, -28.7453) -> (176.842, -28.8456) centre (177.2955, -25.9556) ccw
  arc A336 (175.8816, -28.5559) -> (176.4152, -28.7453) centre (178.8188, -21.128) ccw
  arc A337 (175.3614, -28.3286) -> (175.8816, -28.5559) centre (178.8251, -21.1122) ccw
  arc A338 (174.976, -28.1077) -> (175.3614, -28.3286) centre (176.6802, -25.5808) ccw
  arc A339 (174.7845, -27.9609) -> (174.976, -28.1077) centre (176.088, -26.4589) ccw
  arc A340 (174.5806, -27.7694) -> (174.7845, -27.9609) centre (177.1233, -25.2661) ccw
  arc A341 (174.3897, -27.5598) -> (174.5806, -27.7694) centre (177.1782, -25.212) ccw
  arc A342 (174.2372, -27.3573) -> (174.3897, -27.5598) centre (176.1764, -26.0555) ccw
  arc A343 (174.1623, -27.2364) -> (174.2372, -27.3573) centre (175.859, -26.2686) ccw
  arc A344 (174.0481, -27.0321) -> (174.1623, -27.2364) centre (185.5384, -20.7473) ccw
  arc A345 (173.9215, -26.7954) -> (174.0481, -27.0321) centre (186.9299, -19.9862) ccw
  arc A346 (173.799, -26.5562) -> (173.9215, -26.7954) centre (187.0056, -19.9466) ccw
  line L19 (173.799, -26.5562) -> (173.5072, -25.973)
  line L20 (173.5072, -25.973) -> (173.508, -24.7959)
  arc A347 (173.5198, -23.3765) -> (173.508, -24.7959) centre (267.3598, -24.8638) ccw
  arc A348 (173.5569, -22.3993) -> (173.5198, -23.3765) centre (195.5816, -23.7261) ccw
  arc A349 (173.6217, -21.6946) -> (173.5569, -22.3993) centre (184.7824, -23.0755) ccw
  arc A350 (173.7252, -21.1906) -> (173.6217, -21.6946) centre (176.8371, -22.0924) ccw
  arc A351 (173.9756, -20.6027) -> (173.7252, -21.1906) centre (176.2756, -21.9297) ccw
  arc A352 (174.3734, -20.0488) -> (173.9756, -20.6027) centre (176.95, -22.3188) ccw
  arc A353 (174.8883, -19.5669) -> (174.3734, -20.0488) centre (177.1269, -22.4747) ccw
  arc A354 (175.4855, -19.1928) -> (174.8883, -19.5669) centre (177.1214, -22.4676) ccw
  arc A355 (176.0209, -18.9701) -> (175.4855, -19.1928) centre (177.3576, -22.9403) ccw
  arc A356 (176.6446, -18.7941) -> (176.0209, -18.9701) centre (178.1002, -25.146) ccw
  arc A357 (177.3868, -18.6566) -> (176.6446, -18.7941) centre (178.6532, -27.5593) ccw
  arc A358 (178.2853, -18.5512) -> (177.3868, -18.6566) centre (179.9841, -36.916) ccw
  arc A359 (178.9593, -18.5011) -> (178.2853, -18.5512) centre (180.0122, -37.2196) ccw
  arc A360 (179.4188, -18.5004) -> (178.9593, -18.5011) centre (179.1952, -22.6954) ccw
  arc A361 (179.7833, -18.5478) -> (179.4188, -18.5004) centre (179.2901, -20.9157) ccw
  arc A362 (180.1351, -18.6497) -> (179.7833, -18.5478) centre (179.2961, -20.8869) ccw
  arc A363 (180.4045, -18.7653) -> (180.1351, -18.6497) centre (179.0263, -21.6061) ccw
  arc A364 (180.8558, -18.9899) -> (180.4045, -18.7653) centre (169.5971, -41.0426) ccw
  arc A365 (181.4326, -19.2911) -> (180.8558, -18.9899) centre (164.7577, -50.5217) ccw
  arc A366 (182.1389, -19.6727) -> (181.4326, -19.2911) centre (143.1309, -91.0271) ccw
  line L21 (182.1389, -19.6727) -> (182.9874, -20.1366)
  line L22 (182.9874, -20.1366) -> (184.3771, -19.3478)
  arc A367 (184.9159, -19.0422) -> (184.3771, -19.3478) centre (754.9184, -1024.5156) ccw
  arc A368 (185.384, -18.7771) -> (184.9159, -19.0422) centre (508.4199, -589.6964) ccw
  arc A369 (185.7884, -18.5483) -> (185.384, -18.7771) centre (991.0291, -1442.6331) ccw
  arc A370 (185.8534, -18.5125) -> (185.7884, -18.5483) centre (187.469, -21.5205) ccw
  arc A371 (185.9487, -18.4853) -> (185.8534, -18.5125) centre (185.9635, -18.7176) ccw
  point P0 (100, -50)
  point P1 (132.4837, -36.926)
  constraints: 744 point on circle, 372 centre point, 46 end point
sketch "Sketch18" plane through (-50, 50, 108) normal (0, 0, 1) x (1, 0, 0)
  circle A0 centre (53, -25) radius 11.25
  line L0 (49.2314, -14.4) -> (53.1692, -13)
  line L1 (53.1692, -13) -> (57.0659, -14.5104)
  line L2 (100, -49) -> (100, 0) projected
  line L3 (0, -50) -> (100, -50) projected
  line L4 (108, -49) -> (108, 0) projected
  point P0 (50, -50)
  dimension "d619" = 22.5
  dimension "d621" = 25
  dimension "d628" = 55
  dimension "d629" = 12
  dimension "d631" = 10.6
  constraints: 4 end point, 2 point on circle, 2 tangent, 1 centre point
  measures "d619" diameter of A0
  measures "d621" distance from line of L3 A0.centre
  measures "d628" distance from line of L4 A0.centre
  measures "d629" vertical distance of A0.centre L0.end
  measures "d631" vertical distance of A0.centre L0.start
extrude "Extrusion25" cut sketch "Sketch18" against normal blind 10
mirror "Mirror7" about plane through (0, 0, 0) normal (0, 0, 1) of "Extrusion25"
extrude "Extrusion26" cut sketch "Sketch17" against normal blind 0.8
extrude "Extrusion27" cut sketch "Sketch16" against normal blind 0.8
sketch "Sketch19" plane through (0, 2, 0) normal (0, 1, 0) x (1, 0, 0)
  line L0 (-45, -72.3304) -> (15, -72.3304)
  line L1 (15, -72.3304) -> (15, 67.6696)
  line L2 (15, 67.6696) -> (-45, 67.6696)
  line L3 (-45, 67.6696) -> (-45, -72.3304)
  circle A0 centre (-41, 63.6696) radius 1.55
  circle A1 centre (-41, 63.6696) radius 3
  line L4 (-55, -100) -> (-55, 100) projected
  circle A2 centre (-41, -68.3304) radius 1.55
  circle A3 centre (-41, -68.3304) radius 3
  circle A4 centre (11, -68.3304) radius 1.55
  circle A5 centre (11, -68.3304) radius 3
  circle A6 centre (11, 63.6696) radius 1.55
  circle A7 centre (11, 63.6696) radius 3
  dimension "d632" = 140
  dimension "d633" = 60
  dimension "d637" = 3.1
  dimension "d638" = 4
  dimension "d639" = 4
  dimension "d640" = 6
  dimension "d641" = 10
  dimension "d642" = 3.1
  dimension "d643" = 6
  dimension "d644" = 3.1
  dimension "d645" = 6
  dimension "d646" = 3.1
  dimension "d647" = 6
  dimension "d648" = 4
  dimension "d649" = 4
  dimension "d650" = 4
  dimension "d651" = 4
  dimension "d652" = 4
  dimension "d653" = 4
  constraints: 8 centre point, 8 end point, 4 coincident, 2 parallel, 1 horizontal, 1 perpendicular
  measures "d632" distance of L2.end L0.start
  measures "d633" distance of L1.end L2.end
  measures "d637" diameter of A0
  measures "d638" distance from line of L2 A0.centre
  measures "d639" distance from line of L3 A0.centre
  measures "d640" diameter of A1
  measures "d641" distance between parallel lines of L4 L3
  measures "d642" diameter of A2
  measures "d643" diameter of A3
  measures "d644" diameter of A4
  measures "d645" diameter of A5
  measures "d646" diameter of A6
  measures "d647" diameter of A7
  measures "d648" distance from line of L2 A7.centre
  measures "d649" distance from line of L1 A6.centre
  measures "d650" distance from line of L1 A5.centre
  measures "d651" distance from line of L0 A5.centre
  measures "d652" distance from line of L3 A3.centre
  measures "d653" distance from line of L0 A3.centre
extrude "Extrusion28" add sketch "Sketch19" along normal blind 20 contours A1 | A3 | A5 | A7
